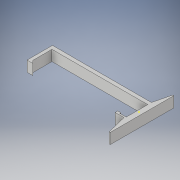
# Autodesk Inventor part: Leg3
Saved by Autodesk Inventor 2019 (Build 230136000, 136)
## iProperties
Created: 2020-04-03
Part Number: Leg3
Material: Generico
Document SubType Name: Modeling
Designer: Administrator
Density: 1 g/cm^3
Appearance: Default
Author: Administrator
Autodesk Inventor part; units mm, degrees
ref_plane "YZ Plane" through (0, 0, 0) normal (1, 0, 0) x (0, 1, 0)
ref_plane "XZ Plane" through (0, 0, 0) normal (0, 1, 0) x (-1, 0, 0)
ref_plane "XY Plane" through (0, 0, 0) normal (0, 0, 1) x (1, 0, 0)
sketch "Sketch1" plane through (0, 0, 0) normal (0, 1, 0) x (-1, 0, 0)
  line L0 (-3, 10) -> (3, 10)
  line L1 (3, 10) -> (3, -10)
  line L2 (3, -10) -> (-3, -10)
  line L3 (-3, -10) -> (-3, 10)
  line L4 (-3, 10) -> (3, -10) construction
  line L5 (3, 10) -> (-3, -10) construction
  line L6 (-3, 10) -> (-3, 30)
  line L7 (-3, 30) -> (-2, 30)
  line L8 (-2, 30) -> (3, 10)
  line L9 (-3, -10) -> (-3, -30)
  line L10 (-3, -30) -> (-2, -30)
  line L11 (-2, -30) -> (3, -10)
  line L12 (-3, 10) -> (3, 10)
  line L13 (3, 10) -> (3, 11.5)
  line L14 (3, 11.5) -> (-3, 11.5)
  line L15 (-3, 11.5) -> (-3, 10)
  line L16 (-3, -10) -> (3, -10)
  line L17 (3, -10) -> (3, -12.5)
  line L18 (3, -12.5) -> (-3, -12.5)
  line L19 (-3, -12.5) -> (-3, -10)
  line L20 (3, 11.5) -> (8, 11.5)
  line L21 (8, 11.5) -> (8, 10)
  line L22 (8, 10) -> (3, 10)
  line L23 (3, 10) -> (3, 11.5)
  line L24 (8, 11.5) -> (11, 11.5)
  line L25 (11, 11.5) -> (11, 9)
  line L26 (11, 9) -> (8, 9)
  line L27 (8, 9) -> (8, 11.5)
  line L28 (3, -10) -> (63, -10)
  line L29 (63, -10) -> (63, -12.5)
  line L30 (63, -12.5) -> (3, -12.5)
  line L31 (3, -12.5) -> (3, -10)
  point P0 (0, 0)
  dimension "d0" = 6
  dimension "d1" = 20
  dimension "d2" = 20
  dimension "d3" = 1
  dimension "d4" = 20
  dimension "d5" = 1
  dimension "d6" = 1.5
  dimension "d7" = 2.5
  dimension "d8" = 5
  dimension "d9" = 3
  dimension "d10" = 2.5
  dimension "d11" = 60
  constraints: 64 end point, 12 parallel, 8 perpendicular, 6 horizontal, 2 midpoint, 1 point on line, 1 vertical
  measures "d0" distance of L1.end L2.end
  measures "d1" distance of L0.end L1.end
  measures "d2" distance of L0.start L6.end
  measures "d3" distance of L6.end L7.end
  measures "d4" distance of L2.end L9.end
  measures "d5" distance of L9.end L10.end
  measures "d6" distance of L13.end L12.end
  measures "d7" distance of L16.end L17.end
  measures "d8" distance of L21.end L22.end
  measures "d9" distance of L25.end L26.end
  measures "d10" distance of L24.end L25.end
  measures "d11" distance of L29.end L30.end
extrude "Extrusion1" add sketch "Sketch1" along normal blind 10
move faces "Move1" translate (1, 0, 0) faces at (-3, 3.3333, -3.3333)
move faces "Move2" translate (0, 0, -0.3) faces at (-22.5833, 6.6667, -12.5) (-42.6667, 3.3333, -10)
move faces "Move3" translate (-29.5, 0, 0) faces at (-63, 3.3333, -11.9667)
move faces "Move4" translate (-2, 0, 0) faces at (-92.5, 3.3333, -11.9667)
sketch "Sketch2" plane through (0, 10, 0) normal (0, 1, 0) x (1, 0, 0)
  point P0 (0, 0)
sketch "Sketch3" plane through (-2, 0, -10.3) normal (0, 0, 1) x (1, 0, 0)
  point P0 (2, 0)
sketch "Sketch4" plane through (-2, 0, -10.3) normal (0, 0, 1) x (1, 0, 0)
  line L0 (-0.3, 0) -> (-92.5, 0) projected
  line L1 (-0.3, 10) -> (-92.5, 10) projected
  line L2 (-92.5, 0) -> (-90.5, 0)
  line L3 (-90.5, 0) -> (-90.5, 10)
  line L4 (-90.5, 10) -> (-92.5, 10)
  line L5 (-92.5, 10) -> (-92.5, 0)
  point P0 (2, 0)
  dimension "d26" = 2
  constraints: 8 end point, 2 parallel, 1 horizontal, 1 perpendicular, 1 point on line
  measures "d26" distance of L4.end L3.end
extrude "Extrusion2" add sketch "Sketch4" along normal blind 15
move faces "Move5" translate (-1, 0, 0) faces at (-94.5, 6.6667, -6.9667)
move faces "Move6" translate (0, 0, 7) faces at (-94.5, 6.6667, 4.7)
sketch "Sketch5" plane through (-92.5, 0, -10.3) normal (1, 0, 0) x (0, 0, -1)
  line L0 (-22, 0) -> (-22, 10) projected
  line L1 (0, 0) -> (-22, 0) projected
  line L2 (-22, 10) -> (-20, 10)
  line L3 (-20, 10) -> (-20, 0)
  line L4 (-20, 0) -> (-22, 0)
  line L5 (-22, 0) -> (-22, 10)
  point P0 (-10.3, 0)
  dimension "d35" = 2
  constraints: 8 end point, 2 parallel, 1 horizontal, 1 perpendicular, 1 point on line
  measures "d35" distance of L3.end L4.end
extrude "Extrusion3" add sketch "Sketch5" along normal blind 2.5
chamfer "Chamfer1" distance 2 angle 45 1 edges at (-92.5, 5, 9.7)
move faces "Move7" translate (0, 0, -2) faces at (-93.6667, 6.6667, 11.7)
move faces "Move8" translate (0, 0, 0.5) faces at (-93.8333, 3.3333, 9.7)
move faces "Move9" translate (0, 0, -1) faces at (-33.3667, 3.3333, -12.8)
body "Solid1"
